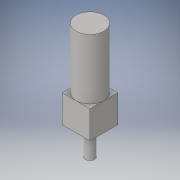
# Autodesk Inventor part: NeveRest motor
Saved by Autodesk Inventor 2016 SP2 (Build 200236200, 236)
## iProperties
Created: 2018-02-13
Part Number: NeveRest motor
Material: Generic
Document SubType Name: Modeling
Designer: CAD
Density: 1 g/cm^3
Appearance: Default
Author: CAD
Autodesk Inventor part; units mm, degrees
ref_plane "YZ Plane" through (0, 0, 0) normal (1, 0, 0) x (0, 1, 0)
ref_plane "XZ Plane" through (0, 0, 0) normal (0, 1, 0) x (-1, 0, 0)
ref_plane "XY Plane" through (0, 0, 0) normal (0, 0, 1) x (1, 0, 0)
sketch "Sketch1" plane through (0, 0, 0) normal (0, 1, 0) x (-1, 0, 0)
  line L0 (0, 0) -> (38.1, 0)
  line L1 (0, 0) -> (0, -38.1)
  line L2 (0, -38.1) -> (38.1, -38.1)
  line L3 (38.1, -38.1) -> (38.1, 0)
  dimension "d0" = 38.1
  dimension "d2" = 38.1
  constraints: 8 end point, 2 horizontal, 1 perpendicular, 1 vertical
  measures "d0" distance of L0.start L0.end
  measures "d2" distance of L0.start L1.end
extrude "Extrusion1" add sketch "Sketch1" along normal blind 38.1
sketch "Sketch2" plane through (0, 38.1, 0) normal (0, 1, 0) x (1, 0, 0)
  circle A0 centre (-19.05, 19.05) radius 19.05
  line L0 (-38.1, 0) -> (-38.1, 38.1) projected
  line L1 (-38.1, 38.1) -> (0, 38.1) projected
  point P0 (0, 0)
  dimension "d5" = 19.05
  dimension "d6" = 19.05
  dimension "d7" = 38.1
  constraints: 1 centre point
  measures "d5" distance from line of L0 A0.centre
  measures "d6" distance from line of L1 A0.centre
  measures "d7" diameter of A0
extrude "Extrusion2" add sketch "Sketch2" along normal blind 82.55 contours A0
sketch "Sketch3" plane through (0, 0, 0) normal (0, -1, 0) x (1, 0, 0)
  circle A0 centre (-19.05, -19.05) radius 6.35
  line L0 (0, -38.1) -> (0, 0) projected
  line L1 (0, 0) -> (-38.1, 0) projected
  dimension "d10" = 12.7
  dimension "d11" = 19.05
  dimension "d12" = 19.05
  constraints: 1 centre point
  measures "d10" diameter of A0
  measures "d11" distance from line of L0 A0.centre
  measures "d12" distance from line of L1 A0.centre
extrude "Extrusion3" add sketch "Sketch3" along normal blind 38.1
body "Solid1"
